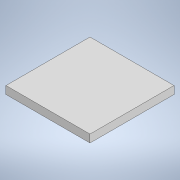
# Autodesk Inventor part: Adapter_Plate_12mm
Saved by Autodesk Inventor 2022.2 (Build 262287010, 287A)
## iProperties
Created: 2024-07-23
Part Number: Adapter_Plate_12mm
Material: Generisch
Document SubType Name: Modeling
Designer: ppovolni
Density: 1 g/cm^3
Appearance: Vorgabe
Author: ppovolni
Autodesk Inventor part; units mm, degrees
ref_plane "YZ Plane" through (0, 0, 0) normal (1, 0, 0) x (0, 1, 0)
ref_plane "XZ Plane" through (0, 0, 0) normal (0, 1, 0) x (-1, 0, 0)
ref_plane "XY Plane" through (0, 0, 0) normal (0, 0, 1) x (1, 0, 0)
sketch "Skizze1" plane through (0, 0, 0) normal (0, 1, 0) x (-1, 0, 0)
  line L0 (-65, -65) -> (65, -65)
  line L1 (65, -65) -> (65, 65)
  line L2 (65, 65) -> (-65, 65)
  line L3 (-65, 65) -> (-65, -65)
  line L4 (-65, -65) -> (65, 65) construction
  line L5 (65, -65) -> (-65, 65) construction
  point P0 (0, 0)
  dimension "d0" = 130
  constraints: 12 end point, 2 midpoint, 2 parallel, 2 perpendicular, 1 horizontal
  measures "d0" distance of L0.end L1.end
extrude "Extrusion1" add sketch "Skizze1" along normal blind 12
